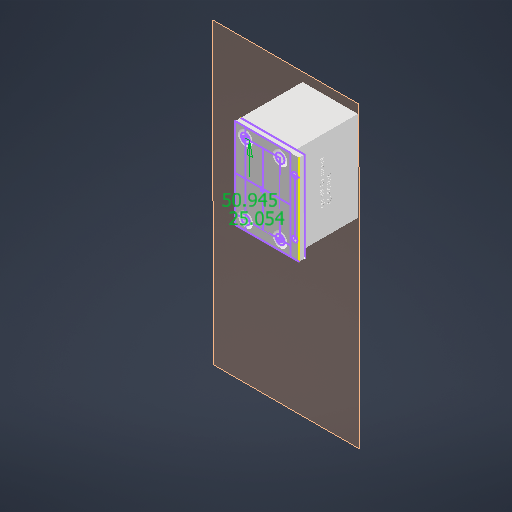
# Autodesk Inventor part: optoNCDT_mount
Saved by Autodesk Inventor 2027 (Build 310192060, 192F)
## iProperties
Created: 2026-05-22
Part Number: optoNCDT_mount
Material: Generic
Document SubType Name: Modeling
Designer: jacob
Density: 1 g/cm^3
Appearance: Default
Author: jacob
Autodesk Inventor part; units mm, degrees
ref_plane "YZ Plane" through (0, 0, 0) normal (1, 0, 0) x (0, 1, 0)
ref_plane "XZ Plane" through (0, 0, 0) normal (0, 1, 0) x (-1, 0, 0)
ref_plane "XY Plane" through (0, 0, 0) normal (0, 0, 1) x (1, 0, 0)
ref_plane "Work Plane2" through (210.6531, -628.7084, 0) normal (0, 0, 1) x (-0.9999994, -0.0010784, 0)
sketch "base_sketch" plane through (210.6531, -628.7084, 0) normal (0, 0, 1) x (-0.9999994, -0.0010784, 0)
  line L0 (229.975, -596.4352) -> (189.975, -596.4352)
  line L1 (189.975, -596.4352) -> (189.975, -661.4352)
  line L2 (189.975, -661.4352) -> (229.975, -661.4352)
  line L3 (229.975, -661.4352) -> (229.975, -596.4352)
  line L4 (209.975, -628.9352) -> (229.975, -628.9352)
  point P0 (209.975, -596.4352)
  dimension "d117" = 65
  dimension "d118" = 40
  constraints: 10 end point, 2 horizontal, 2 midpoint, 2 parallel, 1 perpendicular
  measures "d117" distance of L2.end L0.start
  measures "d118" distance of L1.end L2.end
extrude "base" add sketch "base_sketch" along normal blind 44.8
sketch "top_sketch" plane through (210.6531, -628.7084, 44.8) normal (0, 0, 1) x (0.9999994, 0.0010784, 0)
  line L0 (-229.975, 661.4352) -> (-229.975, 596.4352) projected
  line L1 (-229.975, 596.4352) -> (-183.725, 596.4352)
  line L2 (-183.725, 596.4352) -> (-183.725, 661.4352)
  line L3 (-183.725, 661.4352) -> (-229.975, 661.4352)
  line L4 (-229.975, 661.4352) -> (-229.975, 596.4352)
  line L5 (-189.975, 596.4352) -> (-189.975, 661.4352) projected
  line L6 (-189.975, 661.4352) -> (-229.975, 661.4352)
  point P0 (-209.975, 628.9352)
  point P1 (-228.725, 660.1852)
  point P2 (-229.975, 660.1852)
  constraints: 10 end point, 2 parallel, 1 horizontal, 1 perpendicular
extrude "top" add sketch "top_sketch" along normal blind 4
sketch "label_sketch" plane through (19.9649, 32.5215, 44.8) normal (0.9999994, 0.0010784, 0) x (0, 0, -1)
  line L0 (17.2838, -46.0842) -> (17.2838, 4.2102) construction
  line L1 (17.2838, 4.2102) -> (21.3099, 4.2102) construction
  line L2 (21.3099, 4.2102) -> (21.3099, -46.0842) construction
  line L3 (21.3099, -46.0842) -> (17.2838, -46.0842) construction
  spline S0 degree 2 poles (19.2425, -43.9254) (19.8205, -43.9254) (20.4503, -44.4812) (20.4503, -44.9455) knots 0 0 0 1 2 2 2
  spline S1 degree 2 poles (20.4503, -44.9455) (20.4503, -45.4223) (19.8007, -45.9681) (19.2425, -45.9681) knots 0 0 0 1 2 2 2
  spline S2 degree 2 poles (19.2425, -45.9681) (18.6695, -45.9681) (18.0347, -45.405) (18.0347, -44.9455) knots 0 0 0 1 2 2 2
  spline S3 degree 2 poles (18.0347, -44.9455) (18.0347, -44.4812) (18.667, -43.9254) (19.2425, -43.9254) knots 0 0 0 1 2 2 2
  spline S4 degree 2 poles (19.2425, -44.3231) (18.7979, -44.3231) (18.3656, -44.6467) (18.3656, -44.9455) knots 0 0 0 1 2 2 2
  spline S5 degree 2 poles (18.3656, -44.9455) (18.3656, -45.2444) (18.7979, -45.5705) (19.2425, -45.5705) knots 0 0 0 1 2 2 2
  spline S6 degree 2 poles (19.2425, -45.5705) (19.6747, -45.5705) (20.1193, -45.2444) (20.1193, -44.9455) knots 0 0 0 1 2 2 2
  spline S7 degree 2 poles (20.1193, -44.9455) (20.1193, -44.6491) (19.6822, -44.3231) (19.2425, -44.3231) knots 0 0 0 1 2 2 2
  spline S8 degree 2 poles (19.1807, -41.6135) (19.7538, -41.6135) (20.4306, -42.1594) (20.4306, -42.5768) knots 0 0 0 1 2 2 2
  spline S9 degree 2 poles (20.4306, -42.5768) (20.4306, -42.7472) (20.3515, -43.0091) (20.27, -43.1449) knots 0 0 0 1 2 2 2
  line L4 (20.27, -43.1449) -> (21.2284, -43.1449)
  line L5 (21.2284, -43.1449) -> (21.2284, -43.5302)
  line L6 (21.2284, -43.5302) -> (18.0989, -43.5302)
  line L7 (18.0989, -43.5302) -> (18.0989, -43.1449)
  line L8 (18.0989, -43.1449) -> (18.3385, -43.1449)
  spline S10 degree 2 poles (18.3385, -43.1449) (18.2076, -43.0016) (18.0347, -42.6509) (18.0347, -42.4459) knots 0 0 0 1 2 2 2
  spline S11 degree 2 poles (18.0347, -42.4459) (18.0347, -42.0532) (18.6571, -41.6135) (19.1807, -41.6135) knots 0 0 0 1 2 2 2
  spline S12 degree 2 poles (19.2252, -42.0112) (18.8325, -42.0112) (18.4002, -42.2606) (18.4002, -42.5397) knots 0 0 0 1 2 2 2
  spline S13 degree 2 poles (18.4002, -42.5397) (18.4002, -42.7028) (18.5459, -43.0091) (18.6596, -43.1449) knots 0 0 0 1 2 2 2
  line L9 (18.6596, -43.1449) -> (19.9588, -43.1449)
  spline S14 degree 2 poles (19.9588, -43.1449) (20.0304, -42.9942) (20.0848, -42.7793) (20.0848, -42.641) knots 0 0 0 1 2 2 2
  spline S15 degree 2 poles (20.0848, -42.641) (20.0848, -42.3421) (19.6451, -42.0112) (19.2252, -42.0112) knots 0 0 0 1 2 2 2
  spline S16 degree 2 poles (20.4306, -40.5217) (20.4306, -40.8354) (20.0724, -41.1886) (19.6846, -41.1886) knots 0 0 0 1 2 2 2
  line L10 (19.6846, -41.1886) -> (18.4175, -41.1886)
  line L11 (18.4175, -41.1886) -> (18.4175, -41.448)
  line L12 (18.4175, -41.448) -> (18.0989, -41.448)
  line L13 (18.0989, -41.448) -> (18.0989, -41.1886)
  line L14 (18.0989, -41.1886) -> (17.4419, -41.1886)
  line L15 (17.4419, -41.1886) -> (17.4419, -40.8033)
  line L16 (17.4419, -40.8033) -> (18.0989, -40.8033)
  line L17 (18.0989, -40.8033) -> (18.0989, -40.0944)
  line L18 (18.0989, -40.0944) -> (18.4175, -40.0944)
  line L19 (18.4175, -40.0944) -> (18.4175, -40.8033)
  line L20 (18.4175, -40.8033) -> (19.5068, -40.8033)
  spline S17 degree 2 poles (19.5068, -40.8033) (19.6797, -40.8033) (19.8699, -40.791) (19.9514, -40.749) knots 0 0 0 1 2 2 2
  spline S18 degree 2 poles (19.9514, -40.749) (20.023, -40.7144) (20.0946, -40.5588) (20.0946, -40.4254) knots 0 0 0 1 2 2 2
  spline S19 degree 2 poles (20.0946, -40.4254) (20.0946, -40.3316) (20.0378, -40.1562) (20.0205, -40.1167) knots 0 0 0 1 2 2 2
  line L21 (20.0205, -40.1167) -> (20.0205, -40.0944)
  line L22 (20.0205, -40.0944) -> (20.3664, -40.0944)
  spline S20 degree 2 poles (20.3664, -40.0944) (20.396, -40.2031) (20.4306, -40.4254) (20.4306, -40.5217) knots 0 0 0 1 2 2 2
  spline S21 degree 2 poles (19.2425, -37.9307) (19.8205, -37.9307) (20.4503, -38.4865) (20.4503, -38.9508) knots 0 0 0 1 2 2 2
  spline S22 degree 2 poles (20.4503, -38.9508) (20.4503, -39.4275) (19.8007, -39.9734) (19.2425, -39.9734) knots 0 0 0 1 2 2 2
  spline S23 degree 2 poles (19.2425, -39.9734) (18.6695, -39.9734) (18.0347, -39.4102) (18.0347, -38.9508) knots 0 0 0 1 2 2 2
  spline S24 degree 2 poles (18.0347, -38.9508) (18.0347, -38.4865) (18.667, -37.9307) (19.2425, -37.9307) knots 0 0 0 1 2 2 2
  spline S25 degree 2 poles (19.2425, -38.3284) (18.7979, -38.3284) (18.3656, -38.6519) (18.3656, -38.9508) knots 0 0 0 1 2 2 2
  spline S26 degree 2 poles (18.3656, -38.9508) (18.3656, -39.2497) (18.7979, -39.5757) (19.2425, -39.5757) knots 0 0 0 1 2 2 2
  spline S27 degree 2 poles (19.2425, -39.5757) (19.6747, -39.5757) (20.1193, -39.2497) (20.1193, -38.9508) knots 0 0 0 1 2 2 2
  spline S28 degree 2 poles (20.1193, -38.9508) (20.1193, -38.6544) (19.6822, -38.3284) (19.2425, -38.3284) knots 0 0 0 1 2 2 2
  line L23 (20.3861, -35.3248) -> (20.3861, -35.7793)
  line L24 (20.3861, -35.7793) -> (17.758, -37.1279)
  line L25 (17.758, -37.1279) -> (20.3861, -37.1279)
  line L26 (20.3861, -37.1279) -> (20.3861, -37.5059)
  line L27 (20.3861, -37.5059) -> (17.3381, -37.5059)
  line L28 (17.3381, -37.5059) -> (17.3381, -36.9303)
  line L29 (17.3381, -36.9303) -> (19.7513, -35.7027)
  line L30 (19.7513, -35.7027) -> (17.3381, -35.7027)
  line L31 (17.3381, -35.7027) -> (17.3381, -35.3248)
  line L32 (17.3381, -35.3248) -> (20.3861, -35.3248)
  spline S29 degree 2 poles (20.4405, -33.5168) (20.4405, -33.8132) (20.2404, -34.3146) (20.0403, -34.4974) knots 0 0 0 1 2 2 2
  spline S30 degree 2 poles (20.0403, -34.4974) (19.8427, -34.6802) (19.2499, -34.8802) (18.8646, -34.8802) knots 0 0 0 1 2 2 2
  spline S31 degree 2 poles (18.8646, -34.8802) (18.4817, -34.8802) (17.9136, -34.6851) (17.7037, -34.4998) knots 0 0 0 1 2 2 2
  spline S32 degree 2 poles (17.7037, -34.4998) (17.4987, -34.3171) (17.2838, -33.8181) (17.2838, -33.5094) knots 0 0 0 1 2 2 2
  spline S33 degree 2 poles (17.2838, -33.5094) (17.2838, -33.3562) (17.3282, -33.087) (17.3628, -32.9734) knots 0 0 0 1 2 2 2
  spline S34 degree 2 poles (17.3628, -32.9734) (17.3949, -32.8746) (17.4863, -32.6696) (17.5407, -32.5683) knots 0 0 0 1 2 2 2
  line L33 (17.5407, -32.5683) -> (18.0297, -32.5683)
  line L34 (18.0297, -32.5683) -> (18.0297, -32.6004)
  spline S35 degree 2 poles (18.0297, -32.6004) (17.9803, -32.6547) (17.842, -32.8227) (17.7753, -32.9437) knots 0 0 0 1 2 2 2
  spline S36 degree 2 poles (17.7753, -32.9437) (17.7111, -33.0598) (17.6296, -33.334) (17.6296, -33.5118) knots 0 0 0 1 2 2 2
  spline S37 degree 2 poles (17.6296, -33.5118) (17.6296, -33.707) (17.7901, -34.0552) (17.9433, -34.1862) knots 0 0 0 1 2 2 2
  spline S38 degree 2 poles (17.9433, -34.1862) (18.0989, -34.3146) (18.5706, -34.4579) (18.8646, -34.4579) knots 0 0 0 1 2 2 2
  spline S39 degree 2 poles (18.8646, -34.4579) (19.1783, -34.4579) (19.6303, -34.3072) (19.7859, -34.1763) knots 0 0 0 1 2 2 2
  spline S40 degree 2 poles (19.7859, -34.1763) (19.9366, -34.0478) (20.0897, -33.7045) (20.0897, -33.5118) knots 0 0 0 1 2 2 2
  spline S41 degree 2 poles (20.0897, -33.5118) (20.0897, -33.3365) (20.0033, -33.0376) (19.939, -32.9215) knots 0 0 0 1 2 2 2
  spline S42 degree 2 poles (19.939, -32.9215) (19.8748, -32.8104) (19.7414, -32.6449) (19.6945, -32.5979) knots 0 0 0 1 2 2 2
  line L35 (19.6945, -32.5979) -> (19.6945, -32.5683)
  line L36 (19.6945, -32.5683) -> (20.1786, -32.5683)
  spline S43 degree 2 poles (20.1786, -32.5683) (20.2256, -32.6696) (20.312, -32.8474) (20.3515, -32.9734) knots 0 0 0 1 2 2 2
  spline S44 degree 2 poles (20.3515, -32.9734) (20.396, -33.1068) (20.4405, -33.334) (20.4405, -33.5168) knots 0 0 0 1 2 2 2
  spline S45 degree 2 poles (18.8646, -29.7871) (19.282, -29.7871) (19.9539, -30.1254) (20.1416, -30.4095) knots 0 0 0 1 2 2 2
  spline S46 degree 2 poles (20.1416, -30.4095) (20.2873, -30.6417) (20.3861, -31.1184) (20.3861, -31.4889) knots 0 0 0 1 2 2 2
  line L37 (20.3861, -31.4889) -> (20.3861, -32.1904)
  line L38 (20.3861, -32.1904) -> (17.3381, -32.1904)
  line L39 (17.3381, -32.1904) -> (17.3381, -31.4963)
  spline S47 degree 2 poles (17.3381, -31.4963) (17.3381, -31.0665) (17.4666, -30.5775) (17.5802, -30.4046) knots 0 0 0 1 2 2 2
  spline S48 degree 2 poles (17.5802, -30.4046) (17.7753, -30.1106) (18.42, -29.7871) (18.8646, -29.7871) knots 0 0 0 1 2 2 2
  spline S49 degree 2 poles (18.8596, -30.2094) (18.5089, -30.2094) (18.0124, -30.4416) (17.8716, -30.6713) knots 0 0 0 1 2 2 2
  spline S50 degree 2 poles (17.8716, -30.6713) (17.7753, -30.8343) (17.6889, -31.2024) (17.6889, -31.4765) knots 0 0 0 1 2 2 2
  line L40 (17.6889, -31.4765) -> (17.6889, -31.7853)
  line L41 (17.6889, -31.7853) -> (20.0354, -31.7853)
  line L42 (20.0354, -31.7853) -> (20.0354, -31.4765)
  spline S51 degree 2 poles (20.0354, -31.4765) (20.0354, -31.2073) (19.9489, -30.7998) (19.8328, -30.6343) knots 0 0 0 1 2 2 2
  spline S52 degree 2 poles (19.8328, -30.6343) (19.6896, -30.4218) (19.2153, -30.2094) (18.8596, -30.2094) knots 0 0 0 1 2 2 2
  line L43 (20.3861, -28.636) -> (17.6987, -28.636)
  line L44 (17.6987, -28.636) -> (17.6987, -29.6586)
  line L45 (17.6987, -29.6586) -> (17.3381, -29.6586)
  line L46 (17.3381, -29.6586) -> (17.3381, -27.2084)
  line L47 (17.3381, -27.2084) -> (17.6987, -27.2084)
  line L48 (17.6987, -27.2084) -> (17.6987, -28.2309)
  line L49 (17.6987, -28.2309) -> (20.3861, -28.2309)
  line L50 (20.3861, -28.2309) -> (20.3861, -28.636)
  line L51 (20.3861, -23.0266) -> (19.0622, -23.0266)
  spline S53 degree 2 poles (19.0622, -23.0266) (18.9041, -23.0266) (18.6349, -23.0513) (18.5608, -23.0908) knots 0 0 0 1 2 2 2
  spline S54 degree 2 poles (18.5608, -23.0908) (18.4793, -23.1304) (18.4002, -23.281) (18.4002, -23.4119) knots 0 0 0 1 2 2 2
  spline S55 degree 2 poles (18.4002, -23.4119) (18.4002, -23.5305) (18.5459, -23.8022) (18.6843, -23.9455) knots 0 0 0 1 2 2 2
  spline S56 degree 2 poles (18.6843, -23.9455) (18.7189, -23.943) (18.8152, -23.9381) (18.8794, -23.9381) knots 0 0 0 1 2 2 2
  line L52 (18.8794, -23.9381) -> (20.3861, -23.9381)
  line L53 (20.3861, -23.9381) -> (20.3861, -24.3234)
  line L54 (20.3861, -24.3234) -> (19.0622, -24.3234)
  spline S57 degree 2 poles (19.0622, -24.3234) (18.9041, -24.3234) (18.6349, -24.3481) (18.5608, -24.3876) knots 0 0 0 1 2 2 2
  spline S58 degree 2 poles (18.5608, -24.3876) (18.4793, -24.4271) (18.4002, -24.5778) (18.4002, -24.7087) knots 0 0 0 1 2 2 2
  spline S59 degree 2 poles (18.4002, -24.7087) (18.4002, -24.8322) (18.5558, -25.1064) (18.6769, -25.2348) knots 0 0 0 1 2 2 2
  line L55 (18.6769, -25.2348) -> (20.3861, -25.2348)
  line L56 (20.3861, -25.2348) -> (20.3861, -25.6201)
  line L57 (20.3861, -25.6201) -> (18.0989, -25.6201)
  line L58 (18.0989, -25.6201) -> (18.0989, -25.2348)
  line L59 (18.0989, -25.2348) -> (18.3508, -25.2348)
  spline S60 degree 2 poles (18.3508, -25.2348) (18.2001, -25.0841) (18.0347, -24.7877) (18.0347, -24.6099) knots 0 0 0 1 2 2 2
  spline S61 degree 2 poles (18.0347, -24.6099) (18.0347, -24.4074) (18.2199, -24.0937) (18.4299, -24.0122) knots 0 0 0 1 2 2 2
  spline S62 degree 2 poles (18.4299, -24.0122) (18.2347, -23.8368) (18.0347, -23.5058) (18.0347, -23.3131) knots 0 0 0 1 2 2 2
  spline S63 degree 2 poles (18.0347, -23.3131) (18.0347, -23.1649) (18.126, -22.9229) (18.2298, -22.834) knots 0 0 0 1 2 2 2
  spline S64 degree 2 poles (18.2298, -22.834) (18.3335, -22.7426) (18.6448, -22.6413) (18.8794, -22.6413) knots 0 0 0 1 2 2 2
  line L60 (18.8794, -22.6413) -> (20.3861, -22.6413)
  line L61 (20.3861, -22.6413) -> (20.3861, -23.0266)
  spline S65 degree 2 poles (19.2425, -20.2207) (19.8205, -20.2207) (20.4503, -20.7764) (20.4503, -21.2408) knots 0 0 0 1 2 2 2
  spline S66 degree 2 poles (20.4503, -21.2408) (20.4503, -21.7175) (19.8007, -22.2634) (19.2425, -22.2634) knots 0 0 0 1 2 2 2
  spline S67 degree 2 poles (19.2425, -22.2634) (18.6695, -22.2634) (18.0347, -21.7002) (18.0347, -21.2408) knots 0 0 0 1 2 2 2
  spline S68 degree 2 poles (18.0347, -21.2408) (18.0347, -20.7764) (18.667, -20.2207) (19.2425, -20.2207) knots 0 0 0 1 2 2 2
  spline S69 degree 2 poles (19.2425, -20.6184) (18.7979, -20.6184) (18.3656, -20.9419) (18.3656, -21.2408) knots 0 0 0 1 2 2 2
  spline S70 degree 2 poles (18.3656, -21.2408) (18.3656, -21.5397) (18.7979, -21.8657) (19.2425, -21.8657) knots 0 0 0 1 2 2 2
  spline S71 degree 2 poles (19.2425, -21.8657) (19.6747, -21.8657) (20.1193, -21.5397) (20.1193, -21.2408) knots 0 0 0 1 2 2 2
  spline S72 degree 2 poles (20.1193, -21.2408) (20.1193, -20.9444) (19.6822, -20.6184) (19.2425, -20.6184) knots 0 0 0 1 2 2 2
  line L62 (20.3861, -18.0471) -> (20.3861, -18.4324)
  line L63 (20.3861, -18.4324) -> (20.1342, -18.4324)
  spline S73 degree 2 poles (20.1342, -18.4324) (20.2898, -18.6102) (20.4503, -18.9289) (20.4503, -19.1265) knots 0 0 0 1 2 2 2
  spline S74 degree 2 poles (20.4503, -19.1265) (20.4503, -19.2747) (20.3515, -19.539) (20.2453, -19.6353) knots 0 0 0 1 2 2 2
  spline S75 degree 2 poles (20.2453, -19.6353) (20.1391, -19.7341) (19.8155, -19.8428) (19.5834, -19.8428) knots 0 0 0 1 2 2 2
  line L64 (19.5834, -19.8428) -> (18.0989, -19.8428)
  line L65 (18.0989, -19.8428) -> (18.0989, -19.4574)
  line L66 (18.0989, -19.4574) -> (19.403, -19.4574)
  spline S76 degree 2 poles (19.403, -19.4574) (19.5858, -19.4574) (19.8254, -19.4303) (19.9143, -19.3833) knots 0 0 0 1 2 2 2
  spline S77 degree 2 poles (19.9143, -19.3833) (20.0033, -19.3364) (20.0848, -19.1759) (20.0848, -19.0252) knots 0 0 0 1 2 2 2
  spline S78 degree 2 poles (20.0848, -19.0252) (20.0848, -18.8844) (19.9242, -18.5658) (19.8081, -18.4324) knots 0 0 0 1 2 2 2
  line L67 (19.8081, -18.4324) -> (18.0989, -18.4324)
  line L68 (18.0989, -18.4324) -> (18.0989, -18.0471)
  line L69 (18.0989, -18.0471) -> (20.3861, -18.0471)
  line L70 (20.3861, -15.6931) -> (20.3861, -16.0785)
  line L71 (20.3861, -16.0785) -> (19.0819, -16.0785)
  spline S79 degree 2 poles (19.0819, -16.0785) (18.9239, -16.0785) (18.6522, -16.1081) (18.5706, -16.1526) knots 0 0 0 1 2 2 2
  spline S80 degree 2 poles (18.5706, -16.1526) (18.4842, -16.1995) (18.4002, -16.3675) (18.4002, -16.5107) knots 0 0 0 1 2 2 2
  spline S81 degree 2 poles (18.4002, -16.5107) (18.4002, -16.654) (18.5534, -16.9578) (18.6769, -17.1035) knots 0 0 0 1 2 2 2
  line L72 (18.6769, -17.1035) -> (20.3861, -17.1035)
  line L73 (20.3861, -17.1035) -> (20.3861, -17.4888)
  line L74 (20.3861, -17.4888) -> (18.0989, -17.4888)
  line L75 (18.0989, -17.4888) -> (18.0989, -17.1035)
  line L76 (18.0989, -17.1035) -> (18.3533, -17.1035)
  spline S82 degree 2 poles (18.3533, -17.1035) (18.1977, -16.9306) (18.0347, -16.5972) (18.0347, -16.4094) knots 0 0 0 1 2 2 2
  spline S83 degree 2 poles (18.0347, -16.4094) (18.0347, -16.0735) (18.4793, -15.6931) (18.9016, -15.6931) knots 0 0 0 1 2 2 2
  line L77 (18.9016, -15.6931) -> (20.3861, -15.6931)
  spline S84 degree 2 poles (20.4306, -14.4606) (20.4306, -14.7743) (20.0724, -15.1275) (19.6846, -15.1275) knots 0 0 0 1 2 2 2
  line L78 (19.6846, -15.1275) -> (18.4175, -15.1275)
  line L79 (18.4175, -15.1275) -> (18.4175, -15.3869)
  line L80 (18.4175, -15.3869) -> (18.0989, -15.3869)
  line L81 (18.0989, -15.3869) -> (18.0989, -15.1275)
  line L82 (18.0989, -15.1275) -> (17.4419, -15.1275)
  line L83 (17.4419, -15.1275) -> (17.4419, -14.7422)
  line L84 (17.4419, -14.7422) -> (18.0989, -14.7422)
  line L85 (18.0989, -14.7422) -> (18.0989, -14.0333)
  line L86 (18.0989, -14.0333) -> (18.4175, -14.0333)
  line L87 (18.4175, -14.0333) -> (18.4175, -14.7422)
  line L88 (18.4175, -14.7422) -> (19.5068, -14.7422)
  spline S85 degree 2 poles (19.5068, -14.7422) (19.6797, -14.7422) (19.8699, -14.7298) (19.9514, -14.6878) knots 0 0 0 1 2 2 2
  spline S86 degree 2 poles (19.9514, -14.6878) (20.023, -14.6533) (20.0946, -14.4977) (20.0946, -14.3643) knots 0 0 0 1 2 2 2
  spline S87 degree 2 poles (20.0946, -14.3643) (20.0946, -14.2704) (20.0378, -14.095) (20.0205, -14.0555) knots 0 0 0 1 2 2 2
  line L89 (20.0205, -14.0555) -> (20.0205, -14.0333)
  line L90 (20.0205, -14.0333) -> (20.3664, -14.0333)
  spline S88 degree 2 poles (20.3664, -14.0333) (20.396, -14.142) (20.4306, -14.3643) (20.4306, -14.4606) knots 0 0 0 1 2 2 2
  spline S89 degree 2 poles (24.4166, -43.9353) (24.6512, -43.9353) (25.0489, -44.0909) (25.1823, -44.2218) knots 0 0 0 1 2 2 2
  spline S90 degree 2 poles (25.1823, -44.2218) (25.3231, -44.3577) (25.4688, -44.6985) (25.4688, -44.9036) knots 0 0 0 1 2 2 2
  spline S91 degree 2 poles (25.4688, -44.9036) (25.4688, -45.1086) (25.3305, -45.447) (25.1921, -45.5754) knots 0 0 0 1 2 2 2
  spline S92 degree 2 poles (25.1921, -45.5754) (25.0267, -45.7335) (24.4709, -45.9113) (24.0658, -45.9113) knots 0 0 0 1 2 2 2
  spline S93 degree 2 poles (24.0658, -45.9113) (23.6681, -45.9113) (23.0284, -45.7483) (22.7913, -45.5779) knots 0 0 0 1 2 2 2
  spline S94 degree 2 poles (22.7913, -45.5779) (22.5591, -45.4124) (22.2998, -44.8887) (22.2998, -44.5454) knots 0 0 0 1 2 2 2
  spline S95 degree 2 poles (22.2998, -44.5454) (22.2998, -44.4441) (22.3195, -44.2663) (22.3417, -44.1996) knots 0 0 0 1 2 2 2
  line L91 (22.3417, -44.1996) -> (22.7345, -44.1996)
  line L92 (22.7345, -44.1996) -> (22.7345, -44.2169)
  spline S96 degree 2 poles (22.7345, -44.2169) (22.7048, -44.2737) (22.653, -44.4812) (22.653, -44.5997) knots 0 0 0 1 2 2 2
  spline S97 degree 2 poles (22.653, -44.5997) (22.653, -44.9801) (23.1667, -45.447) (23.6706, -45.4914) knots 0 0 0 1 2 2 2
  spline S98 degree 2 poles (23.6706, -45.4914) (23.5693, -45.3457) (23.4582, -45.0394) (23.4582, -44.8566) knots 0 0 0 1 2 2 2
  spline S99 degree 2 poles (23.4582, -44.8566) (23.4582, -44.6788) (23.5298, -44.412) (23.6385, -44.2663) knots 0 0 0 1 2 2 2
  spline S100 degree 2 poles (23.6385, -44.2663) (23.7645, -44.0983) (24.1547, -43.9353) (24.4166, -43.9353) knots 0 0 0 1 2 2 2
  spline S101 degree 2 poles (24.4338, -44.3503) (24.2461, -44.3503) (23.9917, -44.4491) (23.9028, -44.5578) knots 0 0 0 1 2 2 2
  spline S102 degree 2 poles (23.9028, -44.5578) (23.8386, -44.6393) (23.7966, -44.8418) (23.7966, -44.948) knots 0 0 0 1 2 2 2
  spline S103 degree 2 poles (23.7966, -44.948) (23.7966, -45.0913) (23.883, -45.3605) (23.9645, -45.4914) knots 0 0 0 1 2 2 2
  spline S104 degree 2 poles (23.9645, -45.4914) (24.009, -45.4939) (24.093, -45.4988) (24.1572, -45.4988) knots 0 0 0 1 2 2 2
  spline S105 degree 2 poles (24.1572, -45.4988) (24.4734, -45.4988) (24.8612, -45.3753) (24.9624, -45.2815) knots 0 0 0 1 2 2 2
  spline S106 degree 2 poles (24.9624, -45.2815) (25.0588, -45.195) (25.1353, -45.0073) (25.1353, -44.9011) knots 0 0 0 1 2 2 2
  spline S107 degree 2 poles (25.1353, -44.9011) (25.1353, -44.6541) (24.7846, -44.3503) (24.4338, -44.3503) knots 0 0 0 1 2 2 2
  line L93 (22.2207, -42.3076) -> (26.0665, -43.5006)
  line L94 (26.0665, -43.5006) -> (26.0665, -43.8464)
  line L95 (26.0665, -43.8464) -> (22.2207, -42.6583)
  line L96 (22.2207, -42.6583) -> (22.2207, -42.3076)
  line L97 (25.4046, -40.092) -> (25.4046, -41.9716)
  line L98 (25.4046, -41.9716) -> (24.9723, -41.9716)
  spline S108 degree 2 poles (24.9723, -41.9716) (24.7821, -41.7691) (24.4289, -41.4085) (24.2387, -41.2356) knots 0 0 0 1 2 2 2
  spline S109 degree 2 poles (24.2387, -41.2356) (23.8559, -40.8873) (23.3964, -40.6329) (23.1519, -40.6329) knots 0 0 0 1 2 2 2
  spline S110 degree 2 poles (23.1519, -40.6329) (23.0235, -40.6329) (22.8308, -40.7119) (22.7691, -40.7836) knots 0 0 0 1 2 2 2
  spline S111 degree 2 poles (22.7691, -40.7836) (22.7073, -40.8552) (22.6456, -41.0429) (22.6456, -41.1565) knots 0 0 0 1 2 2 2
  spline S112 degree 2 poles (22.6456, -41.1565) (22.6456, -41.2652) (22.6999, -41.4875) (22.7419, -41.5888) knots 0 0 0 1 2 2 2
  spline S113 degree 2 poles (22.7419, -41.5888) (22.7765, -41.6752) (22.8753, -41.8358) (22.9098, -41.8852) knots 0 0 0 1 2 2 2
  line L99 (22.9098, -41.8852) -> (22.9098, -41.9074)
  line L100 (22.9098, -41.9074) -> (22.4751, -41.9074)
  spline S114 degree 2 poles (22.4751, -41.9074) (22.4134, -41.7815) (22.2923, -41.3294) (22.2923, -41.1269) knots 0 0 0 1 2 2 2
  spline S115 degree 2 poles (22.2923, -41.1269) (22.2923, -40.6996) (22.7444, -40.2179) (23.1297, -40.2179) knots 0 0 0 1 2 2 2
  spline S116 degree 2 poles (23.1297, -40.2179) (23.31, -40.2179) (23.6113, -40.3019) (23.7398, -40.376) knots 0 0 0 1 2 2 2
  spline S117 degree 2 poles (23.7398, -40.376) (23.8732, -40.4501) (24.135, -40.665) (24.2609, -40.7836) knots 0 0 0 1 2 2 2
  spline S118 degree 2 poles (24.2609, -40.7836) (24.4709, -40.9762) (24.9204, -41.448) (25.0514, -41.5888) knots 0 0 0 1 2 2 2
  line L101 (25.0514, -41.5888) -> (25.0514, -40.092)
  line L102 (25.0514, -40.092) -> (25.4046, -40.092)
  line L103 (24.3573, -37.7232) -> (24.3573, -38.0863)
  line L104 (24.3573, -38.0863) -> (25.4046, -38.0863)
  line L105 (25.4046, -38.0863) -> (25.4046, -38.479)
  line L106 (25.4046, -38.479) -> (24.3573, -38.479)
  line L107 (24.3573, -38.479) -> (24.3573, -39.8252)
  line L108 (24.3573, -39.8252) -> (23.9275, -39.8252)
  line L109 (23.9275, -39.8252) -> (22.3566, -38.4618)
  line L110 (22.3566, -38.4618) -> (22.3566, -38.0863)
  line L111 (22.3566, -38.0863) -> (24.0288, -38.0863)
  line L112 (24.0288, -38.0863) -> (24.0288, -37.7232)
  line L113 (24.0288, -37.7232) -> (24.3573, -37.7232)
  line L114 (24.0288, -38.479) -> (22.8382, -38.479)
  line L115 (22.8382, -38.479) -> (24.0288, -39.5041)
  line L116 (24.0288, -39.5041) -> (24.0288, -38.479)
  line L117 (22.2207, -36.1301) -> (26.0665, -37.3231)
  line L118 (26.0665, -37.3231) -> (26.0665, -37.6689)
  line L119 (26.0665, -37.6689) -> (22.2207, -36.4808)
  line L120 (22.2207, -36.4808) -> (22.2207, -36.1301)
  line L121 (25.4046, -33.9145) -> (25.4046, -35.7941)
  line L122 (25.4046, -35.7941) -> (24.9723, -35.7941)
  spline S119 degree 2 poles (24.9723, -35.7941) (24.7821, -35.5916) (24.4289, -35.231) (24.2387, -35.0581) knots 0 0 0 1 2 2 2
  spline S120 degree 2 poles (24.2387, -35.0581) (23.8559, -34.7098) (23.3964, -34.4554) (23.1519, -34.4554) knots 0 0 0 1 2 2 2
  spline S121 degree 2 poles (23.1519, -34.4554) (23.0235, -34.4554) (22.8308, -34.5344) (22.7691, -34.6061) knots 0 0 0 1 2 2 2
  spline S122 degree 2 poles (22.7691, -34.6061) (22.7073, -34.6777) (22.6456, -34.8654) (22.6456, -34.979) knots 0 0 0 1 2 2 2
  spline S123 degree 2 poles (22.6456, -34.979) (22.6456, -35.0877) (22.6999, -35.31) (22.7419, -35.4113) knots 0 0 0 1 2 2 2
  spline S124 degree 2 poles (22.7419, -35.4113) (22.7765, -35.4977) (22.8753, -35.6583) (22.9098, -35.7077) knots 0 0 0 1 2 2 2
  line L123 (22.9098, -35.7077) -> (22.9098, -35.7299)
  line L124 (22.9098, -35.7299) -> (22.4751, -35.7299)
  spline S125 degree 2 poles (22.4751, -35.7299) (22.4134, -35.6039) (22.2923, -35.1519) (22.2923, -34.9494) knots 0 0 0 1 2 2 2
  spline S126 degree 2 poles (22.2923, -34.9494) (22.2923, -34.5221) (22.7444, -34.0404) (23.1297, -34.0404) knots 0 0 0 1 2 2 2
  spline S127 degree 2 poles (23.1297, -34.0404) (23.31, -34.0404) (23.6113, -34.1244) (23.7398, -34.1985) knots 0 0 0 1 2 2 2
  spline S128 degree 2 poles (23.7398, -34.1985) (23.8732, -34.2726) (24.135, -34.4875) (24.2609, -34.6061) knots 0 0 0 1 2 2 2
  spline S129 degree 2 poles (24.2609, -34.6061) (24.4709, -34.7987) (24.9204, -35.2705) (25.0514, -35.4113) knots 0 0 0 1 2 2 2
  line L125 (25.0514, -35.4113) -> (25.0514, -33.9145)
  line L126 (25.0514, -33.9145) -> (25.4046, -33.9145)
  spline S130 degree 2 poles (23.8806, -31.6099) (24.7006, -31.6099) (25.4688, -32.0866) (25.4688, -32.5831) knots 0 0 0 1 2 2 2
  spline S131 degree 2 poles (25.4688, -32.5831) (25.4688, -33.087) (24.6858, -33.5588) (23.883, -33.5588) knots 0 0 0 1 2 2 2
  spline S132 degree 2 poles (23.883, -33.5588) (23.058, -33.5588) (22.2948, -33.0821) (22.2948, -32.5831) knots 0 0 0 1 2 2 2
  spline S133 degree 2 poles (22.2948, -32.5831) (22.2948, -32.0817) (23.0852, -31.6099) (23.8806, -31.6099) knots 0 0 0 1 2 2 2
  spline S134 degree 2 poles (24.8093, -32.1336) (24.6586, -32.0743) (24.1943, -32.0249) (23.8806, -32.0249) knots 0 0 0 1 2 2 2
  spline S135 degree 2 poles (23.8806, -32.0249) (23.5669, -32.0249) (23.105, -32.0743) (22.9494, -32.136) knots 0 0 0 1 2 2 2
  spline S136 degree 2 poles (22.9494, -32.136) (22.7938, -32.1978) (22.6332, -32.4127) (22.6332, -32.5831) knots 0 0 0 1 2 2 2
  spline S137 degree 2 poles (22.6332, -32.5831) (22.6332, -32.7535) (22.7938, -32.9734) (22.9543, -33.0376) knots 0 0 0 1 2 2 2
  spline S138 degree 2 poles (22.9543, -33.0376) (23.1099, -33.0993) (23.5842, -33.1438) (23.883, -33.1438) knots 0 0 0 1 2 2 2
  spline S139 degree 2 poles (23.883, -33.1438) (24.2041, -33.1438) (24.6339, -33.1043) (24.8019, -33.0401) knots 0 0 0 1 2 2 2
  spline S140 degree 2 poles (24.8019, -33.0401) (24.96, -32.9808) (25.1304, -32.761) (25.1304, -32.5831) knots 0 0 0 1 2 2 2
  spline S141 degree 2 poles (25.1304, -32.5831) (25.1304, -32.4152) (24.9698, -32.1953) (24.8093, -32.1336) knots 0 0 0 1 2 2 2
  line L127 (25.4046, -29.34) -> (25.4046, -31.2197)
  line L128 (25.4046, -31.2197) -> (24.9723, -31.2197)
  spline S142 degree 2 poles (24.9723, -31.2197) (24.7821, -31.0171) (24.4289, -30.6565) (24.2387, -30.4836) knots 0 0 0 1 2 2 2
  spline S143 degree 2 poles (24.2387, -30.4836) (23.8559, -30.1353) (23.3964, -29.8809) (23.1519, -29.8809) knots 0 0 0 1 2 2 2
  spline S144 degree 2 poles (23.1519, -29.8809) (23.0235, -29.8809) (22.8308, -29.96) (22.7691, -30.0316) knots 0 0 0 1 2 2 2
  spline S145 degree 2 poles (22.7691, -30.0316) (22.7073, -30.1032) (22.6456, -30.2909) (22.6456, -30.4046) knots 0 0 0 1 2 2 2
  spline S146 degree 2 poles (22.6456, -30.4046) (22.6456, -30.5132) (22.6999, -30.7355) (22.7419, -30.8368) knots 0 0 0 1 2 2 2
  spline S147 degree 2 poles (22.7419, -30.8368) (22.7765, -30.9233) (22.8753, -31.0838) (22.9098, -31.1332) knots 0 0 0 1 2 2 2
  line L129 (22.9098, -31.1332) -> (22.9098, -31.1554)
  line L130 (22.9098, -31.1554) -> (22.4751, -31.1554)
  spline S148 degree 2 poles (22.4751, -31.1554) (22.4134, -31.0295) (22.2923, -30.5775) (22.2923, -30.3749) knots 0 0 0 1 2 2 2
  spline S149 degree 2 poles (22.2923, -30.3749) (22.2923, -29.9476) (22.7444, -29.466) (23.1297, -29.466) knots 0 0 0 1 2 2 2
  spline S150 degree 2 poles (23.1297, -29.466) (23.31, -29.466) (23.6113, -29.5499) (23.7398, -29.624) knots 0 0 0 1 2 2 2
  spline S151 degree 2 poles (23.7398, -29.624) (23.8732, -29.6981) (24.135, -29.913) (24.2609, -30.0316) knots 0 0 0 1 2 2 2
  spline S152 degree 2 poles (24.2609, -30.0316) (24.4709, -30.2242) (24.9204, -30.696) (25.0514, -30.8368) knots 0 0 0 1 2 2 2
  line L131 (25.0514, -30.8368) -> (25.0514, -29.34)
  line L132 (25.0514, -29.34) -> (25.4046, -29.34)
  spline S153 degree 2 poles (24.4166, -27.0058) (24.6512, -27.0058) (25.0489, -27.1614) (25.1823, -27.2923) knots 0 0 0 1 2 2 2
  spline S154 degree 2 poles (25.1823, -27.2923) (25.3231, -27.4282) (25.4688, -27.7691) (25.4688, -27.9741) knots 0 0 0 1 2 2 2
  spline S155 degree 2 poles (25.4688, -27.9741) (25.4688, -28.1791) (25.3305, -28.5175) (25.1921, -28.6459) knots 0 0 0 1 2 2 2
  spline S156 degree 2 poles (25.1921, -28.6459) (25.0267, -28.804) (24.4709, -28.9818) (24.0658, -28.9818) knots 0 0 0 1 2 2 2
  spline S157 degree 2 poles (24.0658, -28.9818) (23.6681, -28.9818) (23.0284, -28.8188) (22.7913, -28.6484) knots 0 0 0 1 2 2 2
  spline S158 degree 2 poles (22.7913, -28.6484) (22.5591, -28.4829) (22.2998, -27.9592) (22.2998, -27.6159) knots 0 0 0 1 2 2 2
  spline S159 degree 2 poles (22.2998, -27.6159) (22.2998, -27.5146) (22.3195, -27.3368) (22.3417, -27.2701) knots 0 0 0 1 2 2 2
  line L133 (22.3417, -27.2701) -> (22.7345, -27.2701)
  line L134 (22.7345, -27.2701) -> (22.7345, -27.2874)
  spline S160 degree 2 poles (22.7345, -27.2874) (22.7048, -27.3442) (22.653, -27.5517) (22.653, -27.6703) knots 0 0 0 1 2 2 2
  spline S161 degree 2 poles (22.653, -27.6703) (22.653, -28.0506) (23.1667, -28.5175) (23.6706, -28.5619) knots 0 0 0 1 2 2 2
  spline S162 degree 2 poles (23.6706, -28.5619) (23.5693, -28.4162) (23.4582, -28.1099) (23.4582, -27.9271) knots 0 0 0 1 2 2 2
  spline S163 degree 2 poles (23.4582, -27.9271) (23.4582, -27.7493) (23.5298, -27.4825) (23.6385, -27.3368) knots 0 0 0 1 2 2 2
  spline S164 degree 2 poles (23.6385, -27.3368) (23.7645, -27.1688) (24.1547, -27.0058) (24.4166, -27.0058) knots 0 0 0 1 2 2 2
  spline S165 degree 2 poles (24.4338, -27.4208) (24.2461, -27.4208) (23.9917, -27.5196) (23.9028, -27.6283) knots 0 0 0 1 2 2 2
  spline S166 degree 2 poles (23.9028, -27.6283) (23.8386, -27.7098) (23.7966, -27.9123) (23.7966, -28.0185) knots 0 0 0 1 2 2 2
  spline S167 degree 2 poles (23.7966, -28.0185) (23.7966, -28.1618) (23.883, -28.431) (23.9645, -28.5619) knots 0 0 0 1 2 2 2
  spline S168 degree 2 poles (23.9645, -28.5619) (24.009, -28.5644) (24.093, -28.5693) (24.1572, -28.5693) knots 0 0 0 1 2 2 2
  spline S169 degree 2 poles (24.1572, -28.5693) (24.4734, -28.5693) (24.8612, -28.4458) (24.9624, -28.352) knots 0 0 0 1 2 2 2
  spline S170 degree 2 poles (24.9624, -28.352) (25.0588, -28.2655) (25.1353, -28.0778) (25.1353, -27.9716) knots 0 0 0 1 2 2 2
  spline S171 degree 2 poles (25.1353, -27.9716) (25.1353, -27.7246) (24.7846, -27.4208) (24.4338, -27.4208) knots 0 0 0 1 2 2 2
  point P0 (44.8, -32.5)
  constraints: 2 other
extrude "label" cut sketch "label_sketch" against normal blind 1
sketch "hole_sketch" plane through (210.6531, -628.7084, 48.8) normal (0, 0, 1) x (0.9999994, 0.0010784, 0)
  circle A0 centre (-222.5019, 603.463) radius 3.25
  circle A1 centre (-197.448, 603.463) radius 3.25
  circle A2 centre (-222.5019, 654.4075) radius 3.25
  circle A3 centre (-197.448, 654.4075) radius 3.25
  line L0 (-229.975, 596.4352) -> (-183.725, 596.4352)
  line L1 (-189.975, 661.4352) -> (-229.975, 661.4352)
  line L2 (-222.5019, 603.463) -> (-197.448, 603.463)
  line L3 (-197.448, 603.463) -> (-197.448, 654.4075)
  line L4 (-197.448, 654.4075) -> (-222.5019, 654.4075)
  line L5 (-222.5019, 654.4075) -> (-222.5019, 603.463)
  line L6 (-222.5019, 603.463) -> (-222.5019, 596.4352)
  line L7 (-222.5019, 654.4075) -> (-222.5019, 661.4352)
  line L8 (-197.448, 603.463) -> (-189.975, 603.463)
  line L9 (-189.975, 596.4352) -> (-189.975, 661.4352)
  line L10 (-222.5019, 603.463) -> (-229.975, 603.463)
  line L11 (-229.975, 661.4352) -> (-229.975, 596.4352)
  line L12 (-222.5019, 628.9352) -> (-197.448, 628.9352)
  line L13 (-209.975, 603.463) -> (-209.975, 654.4075)
  line L14 (-222.5019, 628.9352) -> (-229.975, 628.9352)
  line L15 (-197.448, 628.9352) -> (-189.975, 628.9352)
  circle A4 centre (-186.85, 608.9352) radius 2
  circle A5 centre (-186.85, 648.9352) radius 2
  line L16 (-186.85, 648.9352) -> (-186.85, 608.9352)
  line L17 (-186.85, 648.9352) -> (-183.725, 648.9352)
  line L18 (-183.725, 596.4352) -> (-183.725, 661.4352) projected
  line L19 (-186.85, 648.9352) -> (-189.975, 648.9352)
  point P0 (-209.975, 628.9352)
  dimension "d127" = 25.0539
  dimension "d128" = 50.9445
  constraints: 38 end point, 9 point on line, 6 centre point, 6 midpoint, 3 collinear, 3 horizontal, 3 parallel, 2 coincident, 2 perpendicular
  measures "d127" distance of L2.start L2.end
  measures "d128" distance of L4.end L2.start
hole "medium_hole" at (-12.4995, -25.4858, 48.8) at (-12.5544, 25.4587, 48.8) at (12.4995, 25.4858, 48.8) at (12.5544, -25.4587, 48.8) direction (0, 0, -1) diameter 6.5 end through all
hole "large_hole" at (-12.4995, -25.4858, 48.8) at (12.5544, -25.4587, 48.8) at (12.4995, 25.4858, 48.8) at (-12.5544, 25.4587, 48.8) direction (0, 0, -1) diameter 10.5 depth 21 tip angle 118
hole "small_hole" at (23.1466, -19.975, 48.8) at (23.1034, 20.0249, 48.8) direction (0, 0, -1) diameter 4 end through all
body "Solid2"
